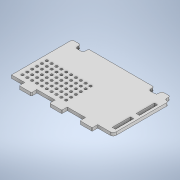
# Autodesk Inventor part: Side_wall
Saved by Autodesk Inventor 2020 (Build 240168000, 168)
## iProperties
Created: 2019-06-12
Part Number: Side_wall
Material: Generic
Document SubType Name: Modeling
Designer: Dammy
Density: 1 g/cm^3
Appearance: Default
Author: Dammy
Autodesk Inventor part; units mm, degrees
ref_plane "YZ Plane" through (0, 0, 0) normal (1, 0, 0) x (0, 1, 0)
ref_plane "XZ Plane" through (0, 0, 0) normal (0, 1, 0) x (-1, 0, 0)
ref_plane "XY Plane" through (0, 0, 0) normal (0, 0, 1) x (1, 0, 0)
sketch "Sketch1" plane through (0, 0, 0) normal (0, 1, 0) x (-1, 0, 0)
  line L0 (80.7, 48.5) -> (80.7, -48.5)
  line L1 (58.95, 48.5) -> (38.95, 48.5)
  line L2 (38.95, 48.5) -> (38.95, 56.5)
  line L3 (39.95, 57.5) -> (57.95, 57.5)
  line L4 (58.95, 56.5) -> (58.95, 48.5)
  line L5 (8.95, 48.5) -> (-11.05, 48.5)
  line L6 (-11.05, 48.5) -> (-11.05, 56.5)
  line L7 (-10.05, 57.5) -> (7.95, 57.5)
  line L8 (8.95, 56.5) -> (8.95, 48.5)
  line L9 (-41.05, 48.5) -> (-61.05, 48.5)
  line L10 (-61.05, 48.5) -> (-61.05, 56.5)
  line L11 (-60.05, 57.5) -> (-42.05, 57.5)
  line L12 (-41.05, 56.5) -> (-41.05, 48.5)
  arc A0 (58.95, 56.5) -> (57.95, 57.5) centre (57.95, 56.5) ccw
  arc A1 (39.95, 57.5) -> (38.95, 56.5) centre (39.95, 56.5) ccw
  arc A2 (8.95, 56.5) -> (7.95, 57.5) centre (7.95, 56.5) ccw
  arc A3 (-10.05, 57.5) -> (-11.05, 56.5) centre (-10.05, 56.5) ccw
  arc A4 (-41.05, 56.5) -> (-42.05, 57.5) centre (-42.05, 56.5) ccw
  arc A5 (-60.05, 57.5) -> (-61.05, 56.5) centre (-60.05, 56.5) ccw
  line L13 (54, -48.5) -> (54, -45.5)
  line L14 (57, -42.5) -> (63.7, -42.5)
  line L15 (66.7, -45.5) -> (66.7, -48.5)
  line L16 (-66.7, -48.5) -> (-66.7, -45.5)
  line L17 (-63.7, -42.5) -> (-57, -42.5)
  line L18 (-54, -45.5) -> (-54, -48.5)
  line L19 (-80.55, -48.5) -> (-80.55, -45.5)
  line L20 (-80.7, 50.1326) -> (10.3, 50.1326) construction
  line L21 (77.7, -51.5) -> (69.7, -51.5)
  line L22 (51, -51.5) -> (-51, -51.5)
  line L23 (-69.7, -51.5) -> (-77.55, -51.5)
  line L24 (-86.55, -39.5) -> (-86.55, 43.5)
  line L25 (80.7, 48.5) -> (-81.55, 48.5)
  line L26 (-83.55, -42.5) -> (-83.55, -42.5)
  arc A6 (77.7, -51.5) -> (80.7, -48.5) centre (77.7, -48.5) ccw
  arc A7 (66.7, -45.5) -> (63.7, -42.5) centre (63.7, -45.5) ccw
  arc A8 (57, -42.5) -> (54, -45.5) centre (57, -45.5) ccw
  arc A9 (51, -51.5) -> (54, -48.5) centre (51, -48.5) ccw
  arc A10 (-54, -48.5) -> (-51, -51.5) centre (-51, -48.5) ccw
  arc A11 (-63.7, -42.5) -> (-66.7, -45.5) centre (-63.7, -45.5) ccw
  arc A12 (-69.7, -51.5) -> (-66.7, -48.5) centre (-69.7, -48.5) ccw
  arc A13 (-80.55, -48.5) -> (-77.55, -51.5) centre (-77.55, -48.5) ccw
  arc A14 (-80.55, -45.5) -> (-83.55, -42.5) centre (-83.55, -45.5) ccw
  arc A15 (66.7, -48.5) -> (69.7, -51.5) centre (69.7, -48.5) ccw
  arc A16 (-54, -45.5) -> (-57, -42.5) centre (-57, -45.5) ccw
  arc A17 (-86.55, -39.5) -> (-83.55, -42.5) centre (-83.55, -39.5) ccw
  arc A18 (-81.55, 48.5) -> (-86.55, 43.5) centre (-81.55, 43.5) ccw
  line L27 (-77.05, -29) -> (-82.3, -29)
  line L28 (-82.3, -29) -> (-82.3, 1)
  line L29 (-82.3, 1) -> (-77.05, 1)
  line L30 (-77.05, 1) -> (-77.05, -29)
  line L31 (-77.05, 10.5) -> (-82.3, 10.5)
  line L32 (-82.3, 10.5) -> (-82.3, 40.5)
  line L33 (-82.3, 40.5) -> (-77.05, 40.5)
  line L34 (-77.05, 40.5) -> (-77.05, 10.5)
  circle A19 centre (71.7, -0.5) radius 2
  circle A20 centre (63.7, -0.5) radius 2
  circle A21 centre (55.7, -0.5) radius 2
  circle A22 centre (47.7, -0.5) radius 2
  circle A23 centre (39.7, -0.5) radius 2
  circle A24 centre (31.7, -0.5) radius 2
  circle A25 centre (23.7, -0.5) radius 2
  circle A26 centre (15.7, -0.5) radius 2
  circle A27 centre (7.7, -0.5) radius 2
  circle A28 centre (-0.3, -0.5) radius 2
  circle A29 centre (71.7, 7.5) radius 2
  circle A30 centre (63.7, 7.5) radius 2
  circle A31 centre (55.7, 7.5) radius 2
  circle A32 centre (47.7, 7.5) radius 2
  circle A33 centre (39.7, 7.5) radius 2
  circle A34 centre (31.7, 7.5) radius 2
  circle A35 centre (23.7, 7.5) radius 2
  circle A36 centre (15.7, 7.5) radius 2
  circle A37 centre (7.7, 7.5) radius 2
  circle A38 centre (-0.3, 7.5) radius 2
  circle A39 centre (71.7, 15.5) radius 2
  circle A40 centre (63.7, 15.5) radius 2
  circle A41 centre (55.7, 15.5) radius 2
  circle A42 centre (47.7, 15.5) radius 2
  circle A43 centre (39.7, 15.5) radius 2
  circle A44 centre (31.7, 15.5) radius 2
  circle A45 centre (23.7, 15.5) radius 2
  circle A46 centre (15.7, 15.5) radius 2
  circle A47 centre (7.7, 15.5) radius 2
  circle A48 centre (-0.3, 15.5) radius 2
  circle A49 centre (71.7, 23.5) radius 2
  circle A50 centre (63.7, 23.5) radius 2
  circle A51 centre (55.7, 23.5) radius 2
  circle A52 centre (47.7, 23.5) radius 2
  circle A53 centre (39.7, 23.5) radius 2
  circle A54 centre (31.7, 23.5) radius 2
  circle A55 centre (23.7, 23.5) radius 2
  circle A56 centre (15.7, 23.5) radius 2
  circle A57 centre (7.7, 23.5) radius 2
  circle A58 centre (-0.3, 23.5) radius 2
  circle A59 centre (71.7, 31.5) radius 2
  circle A60 centre (63.7, 31.5) radius 2
  circle A61 centre (55.7, 31.5) radius 2
  circle A62 centre (47.7, 31.5) radius 2
  circle A63 centre (39.7, 31.5) radius 2
  circle A64 centre (31.7, 31.5) radius 2
  circle A65 centre (23.7, 31.5) radius 2
  circle A66 centre (15.7, 31.5) radius 2
  circle A67 centre (7.7, 31.5) radius 2
  circle A68 centre (-0.3, 31.5) radius 2
  circle A69 centre (71.7, 39.5) radius 2
  circle A70 centre (63.7, 39.5) radius 2
  circle A71 centre (55.7, 39.5) radius 2
  circle A72 centre (47.7, 39.5) radius 2
  circle A73 centre (39.7, 39.5) radius 2
  circle A74 centre (31.7, 39.5) radius 2
  circle A75 centre (23.7, 39.5) radius 2
  circle A76 centre (15.7, 39.5) radius 2
  circle A77 centre (7.7, 39.5) radius 2
  circle A78 centre (-0.3, 39.5) radius 2
  point P0 (0, 0)
  point P1 (80.7, -51.5)
  point P2 (38.95, 57.5)
  point P3 (58.95, 57.5)
  point P4 (51.875, 50)
  point P5 (-11.05, 57.5)
  point P6 (8.95, 57.5)
  point P7 (1.875, 57.5)
  point P8 (-61.05, 57.5)
  point P9 (-41.05, 57.5)
  point P10 (-25.2224, 47.0516)
  point P11 (48.95, 48.5)
  point P12 (-1.05, 48.5)
  point P13 (-51.05, 48.5)
  point P14 (48.95, 57.5)
  point P15 (-1.05, 57.5)
  point P16 (-51.05, 57.5)
  point P17 (66.7, -51.5)
  point P18 (54, -42.5)
  point P19 (54, -51.5)
  point P20 (66.7, -42.5)
  point P21 (-54, -51.5)
  point P22 (-66.7, -42.5)
  point P23 (-66.7, -51.5)
  point P24 (-54, -42.5)
  point P25 (-80.55, -51.5)
  point P26 (-80.55, -42.5)
  point P27 (0, -51.5)
  point P28 (0, 50.1326)
  point P29 (-73.625, -51.5)
  point P30 (73.7, -51.5)
  point P31 (38.95, 48.5)
  point P32 (8.95, 48.5)
  point P33 (-11.05, 48.5)
  point P34 (-41.05, 48.5)
  point P35 (-61.05, 48.5)
  point P36 (80.7, 0)
  dimension "d1" = 100
  dimension "d2" = 21.75
  dimension "d3" = 20
  dimension "d4" = 30
  dimension "d5" = 20
  dimension "d6" = 30
  dimension "d7" = 20
  dimension "d8" = 9
  dimension "d9" = 1
  dimension "d14" = 108
  dimension "d15" = 14
  dimension "d19" = 9
  dimension "d24" = 12.7
  dimension "d25" = 167.25
  dimension "d26" = 3
  dimension "d27" = 3
  dimension "d28" = 3
  dimension "d29" = 12.7
  dimension "d30" = 6
  dimension "d31" = 3
  dimension "d32" = 5
  dimension "d33" = 4.25
  dimension "d34" = 5.25
  dimension "d35" = 30
  dimension "d36" = 9.5
  dimension "d37" = 8
  dimension "d38" = 4
  dimension "d41" = 8
  dimension "d44" = 8
  dimension "d47" = 9
  dimension "d48" = 9
  dimension "d51" = 91
  constraints: 79 centre point, 70 end point, 38 point on circle, 38 tangent, 36 point on line, 15 horizontal alignment, 13 equal radius, 13 horizontal, 13 parallel, 10 midpoint, 7 perpendicular, 3 vertical alignment, 1 collinear, 1 vertical, 118 other
  measures "d1" distance of L0.start point (80.7, -51.5)
  measures "d2" distance between parallel lines of L0 L4
  measures "d3" distance of point (38.95, 57.5) point (58.95, 57.5)
  measures "d4" distance between parallel lines of L2 L8
  measures "d5" distance of point (-11.05, 57.5) point (8.95, 57.5)
  measures "d6" distance between parallel lines of L6 L12
  measures "d7" distance of point (-61.05, 57.5) point (-41.05, 57.5)
  measures "d8" distance between parallel lines of L1 L3
  measures "d9" radius of A0
  measures "d14" distance between parallel lines of L18 L13
  measures "d15" distance between parallel lines of L15 L0
  measures "d19" distance of point (66.7, -51.5) point (66.7, -42.5)
  measures "d24" distance between parallel lines of L13 L15
  measures "d25" distance between parallel lines of L0 L24
  measures "d26" radius of A6
  measures "d27" radius of A15
  measures "d28" radius of A16
  measures "d29" distance of L16.end L18.start
  measures "d30" distance between parallel lines of L24 L19
  measures "d31" radius of A17
  measures "d32" radius of A18
  measures "d33" distance between parallel lines of L24 L28
  measures "d34" distance between parallel lines of L28 L30
  measures "d35" distance between parallel lines of L27 L29
  measures "d36" distance between parallel lines of L31 L29
  measures "d37" distance between parallel lines of L25 L33
  measures "d38" diameter of A19
  measures "d41" distance of A19.centre A20.centre
  measures "d44" distance of A19.centre A29.centre
  measures "d47" distance from line of A69.centre L25
  measures "d48" distance from line of L0 A69.centre
  measures "d51" distance between parallel lines of L25 L14
extrude "Extrusion1" add sketch "Sketch1" along normal blind 5
equation "\"d5\" = d3"
equation "\"d6\" = d4"
equation "\"d7\" = d5"
equation "\"d29\" = d24"
equation "\"d48\" = d47"
body "Solid1"
